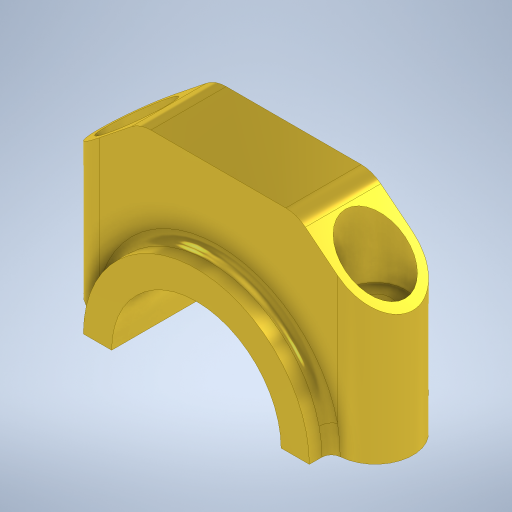
# Autodesk Inventor part: Part4 CONNECTING CAP
Saved by Autodesk Inventor 2023 (Build 270158000, 158)
## iProperties
Created: 2025-10-01
Part Number: Part4 CONNECTING CAP
Material: Stainless Steel
Document SubType Name: Sheet Metal
Designer: ayush
Density: 8 g/cm^3
Sheet Metal Rule: Default_mm
Appearance: Metal 2400F Hot
Author: ayush
Autodesk Inventor part; units mm, degrees
ref_plane "YZ Plane" through (0, 0, 0) normal (1, 0, 0) x (0, 1, 0)
ref_plane "XZ Plane" through (0, 0, 0) normal (0, 1, 0) x (-1, 0, 0)
sketch "Sketch1" plane through (0, 0, 0) normal (0, 0, 1) x (1, 0, 0)
  arc A0 (36, 0) -> (-36, 0) centre (0, 0) ccw
  arc A1 (27, 0) -> (-27, 0) centre (0, 0) ccw
  line L0 (-36, 0) -> (-27, 0)
  line L1 (27, 0) -> (36, 0)
  dimension "d0" = 72
  dimension "d1" = 54
  constraints: 4 end point, 4 point on circle, 2 centre point, 2 coincident, 2 horizontal
  measures "d0" diameter of A0
  measures "d1" diameter of A1
extrude "Extrusion1" add sketch "Sketch1" along normal mid plane 38
ref_plane "Work Plane1" through (27, 60, 19) normal (0, -1, 0) x (1, 0, 0)
sketch "Sketch2" plane through (27, 60, 19) normal (0, -1, 0) x (1, 0, 0)
  line L0 (11, -19) -> (-65, -19) construction
  line L1 (11, -7) -> (-65, -7)
  line L2 (-65, -31) -> (11, -31)
  arc A0 (11, -31) -> (11, -7) centre (11, -19) ccw
  arc A1 (-65, -7) -> (-65, -31) centre (-65, -19) ccw
  line L3 (0, -38) -> (-54, -38) construction
  line L4 (9, 0) -> (9, -38) construction
  point P0 (-27, -19)
  point P1 (-27, -19)
  dimension "d5" = 76
  dimension "d6" = 12
  constraints: 8 end point, 4 point on circle, 4 tangent, 2 centre point, 2 parallel, 1 coincident, 1 midpoint
  measures "d5" distance of L0.start L0.end
  measures "d6" radius of A0
extrude "Extrusion2" add sketch "Sketch2" along normal up to surface (60 mm away)
sketch "Sketch3" plane through (0, 0, 0) normal (0, 0, 1) x (1, 0, 0)
  arc A0 (27, 0) -> (-27, 0) centre (0, 0) ccw projected
  line L0 (27, 0) -> (-27, 0) projected
extrude "Extrusion3" cut sketch "Sketch3" along normal through all both and the other way through all
sketch "Sketch4" plane through (0, 0, 0) normal (0, 0, 1) x (1, 0, 0)
  line L0 (38, 60) -> (-38, 60) projected
  line L1 (-50, 60) -> (-38, 60) projected
  line L2 (-50, 60) -> (-50, 0) projected
  line L3 (-50, 40) -> (-25, 60)
  line L4 (-50, 60) -> (-50, 40)
  point P0 (0, 0)
  dimension "d11" = 25
  dimension "d12" = 20
  constraints: 4 end point, 2 point on line, 1 collinear
  measures "d11" distance of L1.start L3.end
  measures "d12" distance of L1.start L3.start
extrude "Extrusion4" cut sketch "Sketch4" along normal through all both and the other way through all
mirror "Mirror1" about plane through (0, 0, 0) normal (1, 0, 0) of "Extrusion4"
fillet "Fillet1" radius 3 2 edges at (0, 36, -12) (0, 36, 12)
fillet "Fillet2" radius 10 2 edges at (-25, 60, 0) (25, 60, 0)
sketch "Sketch5" plane through (-36, 0, 19) normal (0, -1, 0) x (1, 0, 0)
  arc A0 (-2.8, -7.0267) -> (-2.8, -30.9733) centre (-2, -19) ccw projected
  point P0 (36, -19)
  constraints: 1 coincident
hole "Hole1" at (-38, 0, 0) direction (0, 1, 0) diameter 10 end through all
sketch "Sketch6" plane through (27, 0, -19) normal (0, -1, 0) x (1, 0, 0)
  arc A0 (11.8, 7.0267) -> (11.8, 30.9733) centre (11, 19) ccw projected
  point P0 (-27, 19)
  constraints: 1 coincident
hole "Hole2" at (38, 0, 0) direction (0, 1, 0) diameter 10 end through all
sketch "Sketch7" plane through (27, 60, 19) normal (0, 1, 0) x (1, 0, 0)
  circle A0 centre (-65, 19) radius 5 projected
  circle A1 centre (11, 19) radius 5 projected
  circle A2 centre (-65, 19) radius 5 projected
  point P0 (-27, 19)
  constraints: 2 coincident
hole "Hole3" at (-38, 60, 0) at (38, 60, 0) direction (0, -1, 0) diameter 10 end through all counterbore diameter 19 counterbore depth 25
equation "\"d22\" = Thickness"
equation "\"BendRadius\" = Thickness"
equation "\"BendReliefWidth\" = Thickness"
equation "\"BendReliefDepth\" = 0.5 * Thickness"
equation "\"CornerReliefSize\" = 4 * Thickness"
equation "\"MinimumRemnant\" = 2 * Thickness"
equation "\"TransitionRadius\" = BendRadius"
equation "\"JacobiRadiusSize\" = BendRadius"
equation "\"GapSize\" = Thickness"
equation "\"Thickness\" = 0.5"
body "Solid1"
